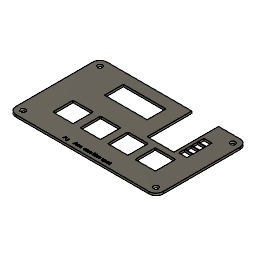
Fullybuiltcase (Autodesk Fusion 360 archive; units mm, degrees)
design "Keycaps"
part number: 2025-11-30-01-42-58-661
Autodesk Fusion 360 part; units mm, degrees
sketch "Sketch3" plane through (0, 0, 0) normal (0, 0, 1) x (1, 0, 0)
  line L0 (16.717, -34.87) -> (29.717, -34.87)
  line L1 (16.717, -48.87) -> (29.717, -48.87)
  line L2 (16.217, -35.37) -> (16.217, -48.37)
  line L3 (30.217, -35.37) -> (30.217, -48.37)
  arc A0 (16.717, -34.87) -> (16.217, -35.37) centre (16.717, -35.37) ccw
  arc A1 (30.217, -35.37) -> (29.717, -34.87) centre (29.717, -35.37) ccw
  arc A2 (16.217, -48.37) -> (16.717, -48.87) centre (16.717, -48.37) ccw
  arc A3 (29.717, -48.87) -> (30.217, -48.37) centre (29.717, -48.37) ccw
  line L4 (35.767, -34.87) -> (48.767, -34.87)
  line L5 (35.767, -48.87) -> (48.767, -48.87)
  line L6 (35.267, -35.37) -> (35.267, -48.37)
  line L7 (49.267, -35.37) -> (49.267, -48.37)
  arc A4 (35.767, -34.87) -> (35.267, -35.37) centre (35.767, -35.37) ccw
  arc A5 (49.267, -35.37) -> (48.767, -34.87) centre (48.767, -35.37) ccw
  arc A6 (35.267, -48.37) -> (35.767, -48.87) centre (35.767, -48.37) ccw
  arc A7 (48.767, -48.87) -> (49.267, -48.37) centre (48.767, -48.37) ccw
  line L8 (54.817, -34.87) -> (67.817, -34.87)
  line L9 (54.817, -48.87) -> (67.817, -48.87)
  line L10 (54.317, -35.37) -> (54.317, -48.37)
  line L11 (68.317, -35.37) -> (68.317, -48.37)
  arc A8 (54.817, -34.87) -> (54.317, -35.37) centre (54.817, -35.37) ccw
  arc A9 (68.317, -35.37) -> (67.817, -34.87) centre (67.817, -35.37) ccw
  arc A10 (54.317, -48.37) -> (54.817, -48.87) centre (54.817, -48.37) ccw
  arc A11 (67.817, -48.87) -> (68.317, -48.37) centre (67.817, -48.37) ccw
  line L12 (73.867, -34.87) -> (86.867, -34.87)
  line L13 (73.867, -48.87) -> (86.867, -48.87)
  line L14 (73.367, -35.37) -> (73.367, -48.37)
  line L15 (87.367, -35.37) -> (87.367, -48.37)
  arc A12 (73.867, -34.87) -> (73.367, -35.37) centre (73.867, -35.37) ccw
  arc A13 (87.367, -35.37) -> (86.867, -34.87) centre (86.867, -35.37) ccw
  arc A14 (73.367, -48.37) -> (73.867, -48.87) centre (73.867, -48.37) ccw
  arc A15 (86.867, -48.87) -> (87.367, -48.37) centre (86.867, -48.37) ccw
  line L16 (0, 0) -> (102.43, 0)
  line L17 (102.43, 0) -> (102.43, -63.37)
  line L18 (102.43, -63.37) -> (0, -63.37)
  line L19 (0, -63.37) -> (0, 0)
  line L20 (63.932, 0) -> (82.432, 0)
  line L21 (82.432, 0) -> (82.432, -31)
  line L22 (82.432, -31) -> (63.932, -31)
  line L23 (63.932, -31) -> (63.932, 0)
  line L24 (84.57, -25.722) -> (90.17, -25.722)
  line L25 (90.17, -25.722) -> (90.17, -29.722)
  line L26 (90.17, -29.722) -> (84.57, -29.722)
  line L27 (84.57, -29.722) -> (84.57, -25.722)
  line L28 (84.57, -21.25) -> (90.17, -21.25)
  line L29 (90.17, -21.25) -> (90.17, -25.25)
  line L30 (90.17, -25.25) -> (84.57, -25.25)
  line L31 (84.57, -25.25) -> (84.57, -21.25)
  line L32 (84.57, -16.777) -> (90.17, -16.777)
  line L33 (90.17, -16.777) -> (90.17, -20.777)
  line L34 (90.17, -20.777) -> (84.57, -20.777)
  line L35 (84.57, -20.777) -> (84.57, -16.777)
  line L36 (84.57, -12.305) -> (90.17, -12.305)
  line L37 (90.17, -12.305) -> (90.17, -16.305)
  line L38 (90.17, -16.305) -> (84.57, -16.305)
  line L39 (84.57, -16.305) -> (84.57, -12.305)
  line L40 (24.102, -7.785) -> (53.602, -7.785)
  line L41 (53.602, -7.785) -> (53.602, -20.785)
  line L42 (53.602, -20.785) -> (24.102, -20.785)
  line L43 (24.102, -20.785) -> (24.102, -7.785)
  circle A16 centre (5, -5) radius 1.7
  circle A17 centre (97.43, -5) radius 1.7
  circle A18 centre (97.43, -58.37) radius 1.7
  circle A19 centre (5, -58.37) radius 1.7
  line L44 (27.3365, -63.37) -> (75.0935, -63.37) construction
  line L45 (75.0935, -63.37) -> (75.0935, -56.3595) construction
  line L46 (75.0935, -56.3595) -> (27.3365, -56.3595) construction
  line L47 (27.3365, -56.3595) -> (27.3365, -63.37) construction
  dimension "d22" = 102.43
  dimension "d23" = 63.37
  dimension "d25" = 14
  dimension "d26" = 14
  dimension "d32" = 5.05
  dimension "d33" = 5.05
  dimension "d34" = 5.05
  dimension "d35" = 14
  dimension "d36" = 14
  dimension "d37" = 14
  dimension "d38" = 14
  dimension "d39" = 14
  dimension "d40" = 14
  dimension "d44" = 63.932
  dimension "d46" = 18.5
  dimension "d47" = 31
  dimension "d52" = 5.6
  dimension "d53" = 4
  dimension "d54" = 5.6
  dimension "d55" = 4
  dimension "d56" = 4
  dimension "d57" = 5.6
  dimension "d58" = 4
  dimension "d59" = 5.6
  dimension "d61" = 29.5
  dimension "d64" = 3.4
  dimension "d65" = 3.4
  dimension "d66" = 3.4
  dimension "d67" = 3.4
  dimension "d68" = 5
  dimension "d69" = 5
  dimension "d70" = 5
  dimension "d71" = 5
  dimension "d72" = 5
  dimension "d73" = 5
  dimension "d74" = 5
  dimension "d75" = 5
  dimension "d80" = 2
  dimension "d87" = 16.217
  dimension "d88" = 14.5
  dimension "d96" = 18.3848
  dimension "d97" = 18.3848
  dimension "d98" = 18.3848
  dimension "d99" = 18.3848
  dimension "d100" = 18.3848
  dimension "d101" = 18.3848
  dimension "d102" = 18.3848
  dimension "d103" = 18.3848
  dimension "d104" = 6.05
  dimension "d105" = 6.05
  dimension "d106" = 6.05
  dimension "d107" = 6.05
  dimension "d108" = 6.05
  dimension "d109" = 0.5
  dimension "d110" = 0.5
  dimension "d111" = 0.5
  dimension "d112" = 0.5
  dimension "d113" = 0.5
  dimension "d114" = 0.5
  dimension "d115" = 0.5
  dimension "d116" = 0.5
  dimension "d117" = 0.5
  dimension "d118" = 0.5
  dimension "d119" = 0.5
  dimension "d120" = 0.5
  dimension "d121" = 0.5
  dimension "d122" = 0.5
  dimension "d123" = 0.5
  dimension "d124" = 0.5
  dimension "d125" = 84.57
  dimension "d126" = 33.648
  dimension "d127" = 38.12
  dimension "d128" = 84.57
  dimension "d129" = 42.593
  dimension "d130" = 84.57
  dimension "d131" = 47.065
  dimension "d132" = 84.57
  text T0 "Arjun Awesome Macropad" font "Arial" height 2 align centre middle in box 47.7571 x 7.0105 at (27.3365, -63.37) x (1, 0) y (0, 1) spacing 1 kerned
  constraint horizontal L16
  constraint vertical L17
  constraint horizontal L18
  constraint vertical L19
  constraint coincident L16.start L19.end
  constraint horizontal L20
  constraint vertical L21
  constraint horizontal L22
  constraint vertical L23
  constraint coincident L16 L20.start
  constraint horizontal L24
  constraint vertical L25
  constraint horizontal L26
  constraint vertical L27
  constraint horizontal L40
  constraint vertical L41
  constraint horizontal L42
  constraint vertical L43
  constraint horizontal L44
  constraint midpoint L18 L44
  measures "d22" distance of L16.start L16.end
  measures "d23" distance of L16.end L17.end
  measures "d25" distance of L2 L3
  measures "d26" distance of L0 L1
  measures "d32" distance of L7 L10
  measures "d33" distance of L11 L14
  measures "d34" distance of L3 L6
  measures "d35" distance of L4 L5
  measures "d36" distance of L6 L7
  measures "d37" distance of L10 L11
  measures "d38" distance of L8 L9
  measures "d39" distance of L14 L15
  measures "d40" distance of L12 L13
  measures "d44" distance of L19 L23
  measures "d46" distance of L21 L23
  measures "d47" distance of L20 L22
  measures "d52" distance of L25 L27
  measures "d53" distance of L24 L26
  measures "d54" distance of L29 L31
  measures "d55" distance of L28 L30
  measures "d56" distance of L32 L34
  measures "d57" distance of L33 L35
  measures "d58" distance of L36 L38
  measures "d59" distance of L37 L39
  measures "d61" distance of L41 L43
  measures "d64" diameter of A16
  measures "d65" diameter of A17
  measures "d66" diameter of A18
  measures "d67" diameter of A19
  measures "d68" distance of L18 A19.centre
  measures "d69" distance of L19 A19.centre
  measures "d70" distance of L16 A16.centre
  measures "d71" distance of L19 A16.centre
  measures "d72" distance of L18 A18.centre
  measures "d73" distance of L17 A18.centre
  measures "d74" distance of L17 A17.centre
  measures "d75" distance of L16 A17.centre
  measures "d87" distance of L2 L19
  measures "d88" distance of L1 L18
  measures "d96" distance of A0.centre A3.centre
  measures "d97" distance of A1.centre A2.centre
  measures "d98" distance of A4.centre A7.centre
  measures "d99" distance of A5.centre A6.centre
  measures "d100" distance of A8.centre A11.centre
  measures "d101" distance of A9.centre A10.centre
  measures "d102" distance of A12.centre A15.centre
  measures "d103" distance of A13.centre A14.centre
  measures "d104" distance of A3.centre A6.centre
  measures "d105" distance of A1.centre A4.centre
  measures "d106" distance of A5.centre A8.centre
  measures "d107" distance of A9.centre A12.centre
  measures "d108" horizontal distance of A11.centre L13.start
  measures "d109" radius of A2
  measures "d110" radius of A0
  measures "d111" radius of A1
  measures "d112" radius of A3
  measures "d113" radius of A6
  measures "d114" radius of A4
  measures "d115" radius of A5
  measures "d116" radius of A7
  measures "d117" radius of A10
  measures "d118" radius of A8
  measures "d119" radius of A9
  measures "d120" radius of A11
  measures "d121" radius of A14
  measures "d122" radius of A12
  measures "d123" radius of A13
  measures "d124" radius of A15
  measures "d125" distance of L19 L27
  measures "d126" distance of L18 L26
  measures "d127" distance of L18 L30
  measures "d128" distance of L19 L31
  measures "d129" distance of L18 L34
  measures "d130" distance of L19 L35
  measures "d131" distance of L18 L38
  measures "d132" distance of L19 L39
sketch "Sketch4" plane through (0, 0, 0) normal (0, 0, 1) x (1, 0, 0)
extrude "Extrude4" add sketch "Sketch3" along normal blind 1.5 contours L16 L17 L18 L19 L21 L22 L23 makes body 1
extrude "Extrude5" add sketch "Sketch3" against normal blind 0.2 from surface at 1.5 separate body text T0 makes body 2 at (37.1638, -60.1289, 1.5) makes body 3 at (38.1775, -60.4327, 1.5) makes body 4 at (40.2716, -60.118, 1.5) makes body 5 at (44.3121, -60.1776, 1.5) makes body 6 at (48.4194, -60.1183, 1.5) makes body 7 at (49.1476, -60.0402, 1.5) makes body 8 at (53.8351, -60.1358, 1.5) makes body 9 at (58.7754, -60.4534, 1.5) makes body 10 at (60.7164, -60.1289, 1.5) makes body 11 at (63.1983, -60.377, 1.5) makes body 12 at (65.7645, -60.4534, 1.5) makes body 13 at (61.5678, -60.0402, 1.5) makes body 14 at (59.3597, -60.5787, 1.5) makes body 15 at (57.2057, -59.6401, 1.5) makes body 16 at (50.7832, -60.1312, 1.5) makes body 17 at (67.32, -59.9124, 1.5) makes body 18 at (47.0029, -60.1358, 1.5) makes body 19 at (43.5708, -59.9243, 1.5) makes body 20 at (39.7232, -60.1576, 1.5) makes body 21 at (38.1775, -59.0548, 1.5) makes body 22 at (36.4262, -59.9243, 1.5)
fillet "Fillet2" radius 5 4 edges at (102.43, 0, 0.75) (102.43, -63.37, 0.75) (0, -63.37, 0.75) (0, 0, 0.75) on bodies 1
equation "d81 = 'Arjun Awesome Macropad'"

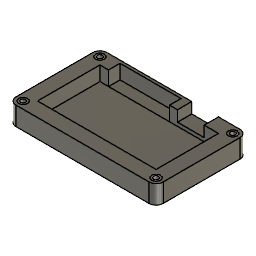
design "BottomCase"
part number: 2025-11-30-01-11-39-605
part number: 2025-11-30-01-15-20-144
Autodesk Fusion 360 part; units mm, degrees
sketch "Sketch1" plane through (0, 0, 0) normal (0, 0, 1) x (1, 0, 0) in component "Arjun's Awesome Macropad"
  line L0 (-41, 23) -> (41.43, 23)
  line L1 (41.43, 23) -> (41.43, -20.37)
  line L2 (41.43, -20.37) -> (-41, -20.37)
  line L3 (-41, -20.37) -> (-41, 23)
  line L4 (-51, 33) -> (51.43, 33)
  line L5 (51.43, 33) -> (51.43, -30.37)
  line L6 (51.43, -30.37) -> (-51, -30.37)
  line L7 (-51, -30.37) -> (-51, 33)
  circle A0 centre (-46, -25.37) radius 1.7
  circle A1 centre (-46, 28) radius 1.7
  circle A2 centre (46.43, -25.37) radius 1.7
  circle A3 centre (46.43, 28) radius 1.7
  circle A4 centre (-46, 28) radius 3
  circle A5 centre (-46, -25.37) radius 3
  circle A6 centre (46.43, 28) radius 3
  circle A7 centre (46.43, -25.37) radius 3
  dimension "d1" = 82.43
  dimension "d2" = 43.37
  dimension "d3" = 10
  dimension "d4" = 10
  dimension "d5" = 10
  dimension "d6" = 10
  dimension "d7" = 3.4
  dimension "d8" = 5
  dimension "d9" = 5
  dimension "d10" = 5
  dimension "d11" = 5
  dimension "d12" = 3.4
  dimension "d13" = 3.4
  dimension "d14" = 5
  dimension "d15" = 5
  dimension "d16" = 5
  dimension "d17" = 5
  dimension "d18" = 3.4
  dimension "d19" = 6
  dimension "d20" = 6
  dimension "d21" = 6
  dimension "d22" = 6
  constraint horizontal L0
  constraint vertical L1
  constraint horizontal L2
  constraint vertical L3
  constraint horizontal L4
  constraint vertical L5
  constraint horizontal L6
  constraint vertical L7
  constraint coincident A1.centre A4.centre
  constraint coincident A0.centre A5.centre
  constraint coincident A3.centre A6.centre
  constraint coincident A2.centre A7.centre
  measures "d1" distance of L0.start L0.end
  measures "d2" distance of L0.end L1.end
  measures "d3" distance of L0.start L7
  measures "d4" distance of L0.end L5
  measures "d5" distance of L2 L6
  measures "d6" distance of L0 L4
  measures "d7" diameter of A0
  measures "d8" distance of L6 A0.centre
  measures "d9" distance of L7 A0.centre
  measures "d10" distance of L4 A1.centre
  measures "d11" distance of L7 A1.centre
  measures "d12" diameter of A1
  measures "d13" diameter of A2
  measures "d14" distance of L6 A2.centre
  measures "d15" distance of L5 A2.centre
  measures "d16" distance of L5 A3.centre
  measures "d17" distance of L4 A3.centre
  measures "d18" diameter of A3
  measures "d19" diameter of A4
  measures "d20" diameter of A5
  measures "d21" diameter of A6
  measures "d22" diameter of A7
extrude "Extrude1" add sketch "Sketch1" along normal blind 9.9 from surface at 3.1 contours A4 | A5 | A6 | A7 makes body 1 at (49.4263, 27.8505, 9.7) makes body 2 at (49.4263, -25.5195, 9.7) makes body 3 at (-43.0037, 27.8505, 9.7) makes body 4 at (-43.0037, -25.5195, 9.7) in component "Arjun's Awesome Macropad"
extrude "Extrude2" add sketch "Sketch1" along normal blind 13 separate body contours L4 L5 L6 L7 makes body 5 in component "Arjun's Awesome Macropad"
extrude "Extrude3" add sketch "Sketch1" along normal blind 3 separate body contours L0 L1 L2 L3 makes body 6 in component "Arjun's Awesome Macropad"
sketch "Sketch2" plane through (0, 0, 13) normal (0, 0, 1) x (-1, 0, 0) in component "Arjun's Awesome Macropad"
  line L0 (-41.43, 20.37) -> (41, 20.37)
  line L1 (41, 20.37) -> (41, -23)
  line L2 (41, -23) -> (-41.43, -23)
  line L3 (-41.43, -23) -> (-41.43, 20.37)
  circle A0 centre (-46.43, 25.37) radius 3
  circle A1 centre (46, -28) radius 3
  circle A2 centre (-46.43, -28) radius 3
  circle A3 centre (46, 25.37) radius 3
  line L4 (51, 30.37) -> (-51.43, 30.37)
  line L5 (-51.43, 30.37) -> (-51.43, -33)
  line L6 (-51.43, -33) -> (51, -33)
  line L7 (51, -33) -> (51, 30.37)
  line L8 (-12.932, -33) -> (-31.432, -33)
  line L9 (-31.432, -33) -> (-31.432, -23)
  line L10 (-31.432, -23) -> (-12.932, -23)
  line L11 (-12.932, -23) -> (-12.932, -33)
  line L12 (51, 30.37) -> (51, -33)
  line L13 (35, -31) -> (-7.415, -31)
  line L14 (-7.415, -31) -> (-7.415, -23)
  line L15 (-7.415, -23) -> (35, -23)
  line L16 (35, -23) -> (35, -31)
  dimension "d31" = 63.932
  dimension "d32" = 18.5
  constraint horizontal L8
  constraint vertical L9
  constraint horizontal L10
  constraint vertical L11
  constraint coincident L2 L9.end
  constraint coincident L6 L8.start
  constraint horizontal L13
  constraint vertical L14
  constraint horizontal L15
  constraint vertical L16
  constraint coincident L2 L14.end
  measures "d31" distance of L11 L12
  measures "d32" distance of L9 L11
extrude "Extrude4" cut sketch "Sketch2" against normal blind 7.5 contours L2 L6 L8 L9 L10 L11 bodies 5 in component "Arjun's Awesome Macropad"
fillet "Fillet1" radius 5 4 edges at (-51, 33, 6.5) (-51, -30.37, 6.5) (51.43, -30.37, 6.5) (51.43, 33, 6.5) on bodies 5 in component "Arjun's Awesome Macropad"
extrude "Extrude5" cut sketch "Sketch2" against normal blind 10 contours L2 L13 L14 L15 L16 bodies 5 in component "Arjun's Awesome Macropad"
component "Arjun's Awesome Macropad" placed x (1, 0, 0) y (0, 1, 0) z (0, 0, 1) at (0, 0, 0)
